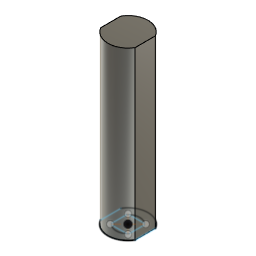
Joystick Extender (Autodesk Fusion 360 design; units mm, degrees)
Autodesk Fusion 360 part; units mm, degrees
sketch "Sketch1" plane through (0, 0, 0) normal (0, 0, 1) x (1, 0, 0)
  line L0 (1.3229, -1.5) -> (-1.3229, -1.5)
  line L1 (-1.5, -1.3229) -> (-1.5, 1.3229)
  line L2 (-1.3229, 1.5) -> (1.3229, 1.5)
  line L3 (1.5, 1.3229) -> (1.5, -1.3229)
  line L4 (1.5, -1.5) -> (-1.5, 1.5) construction
  line L5 (-1.5, -1.5) -> (1.5, 1.5) construction
  arc A0 (-1.5, -1.3229) -> (1.5, -1.3229) centre (0, 0) ccw
  arc A1 (1.5, 1.3229) -> (-1.5, 1.3229) centre (0, 0) ccw
  line L6 (-3, -1.8028) -> (-3, 1.8028)
  arc A2 (3, 1.8028) -> (-3, 1.8028) centre (0, 0) ccw
  line L7 (3, 1.8028) -> (3, -1.8028)
  arc A3 (-3, -1.8028) -> (3, -1.8028) centre (0, 0) ccw
  dimension "d1" = 4
  dimension "d2" = 3
  dimension "d3" = 3
  dimension "d4" = 1.5
  constraint coincident A0.centre A1.centre
  constraint horizontal L0
  constraint perpendicular L0 L1
  constraint parallel L0 L2
  constraint parallel L1 L3
  constraint coincident L4 A0.centre
  constraint coincident L5 A0.centre
  constraint coincident L2.start A0
  constraint coincident L0.end A0
  constraint coincident L3.start A0
  constraint coincident L2.end A0
  constraint coincident L0.start A0
  constraint concentric A0 A1
  measures "d1" diameter of A0
  measures "d2" distance of L4.end L5.end
  measures "d3" distance of L5.start L4.end
extrude "Extrude1" add sketch "Sketch1" along normal blind 30 contours L0 A0 | L0 L1 L2 L3 A0 A1 | L2 A1 | L6 A2 L7 A3 makes body 1
extrude "Extrude2" cut sketch "Sketch1" along normal blind 5 contours L0 A0 | L0 L1 L2 L3 A0 A1 | L2 A1 bodies 1
sketch "Sketch2" plane through (0, 0, 0) normal (0, 0, 1) x (1, 0, 0)
  line L0 (1.3601, -1.6) -> (-1.3601, -1.6)
  line L1 (-1.6, -1.3601) -> (-1.6, 1.3601)
  line L2 (-1.3601, 1.6) -> (1.3601, 1.6)
  line L3 (1.6, 1.3601) -> (1.6, -1.3601)
  line L4 (1.6, -1.6) -> (-1.6, 1.6) construction
  line L5 (-1.6, -1.6) -> (1.6, 1.6) construction
  arc A0 (-1.6, -1.3601) -> (1.6, -1.3601) centre (0, 0) ccw
  arc A1 (1.6, 1.3601) -> (-1.6, 1.3601) centre (0, 0) ccw
  line L6 (-3.1, -1.8303) -> (-3.1, 1.8303)
  arc A2 (3.1, 1.8303) -> (-3.1, 1.8303) centre (0, 0) ccw
  line L7 (3.1, 1.8303) -> (3.1, -1.8303)
  arc A3 (-3.1, -1.8303) -> (3.1, -1.8303) centre (0, 0) ccw
  dimension "d9" = 4.2
  dimension "d10" = 3.2
  dimension "d11" = 3.2
  dimension "d12" = 1.5
  constraint coincident A0.centre A1.centre
  constraint horizontal L0
  constraint perpendicular L0 L1
  constraint parallel L0 L2
  constraint parallel L1 L3
  constraint coincident L4 A0.centre
  constraint coincident L5 A0.centre
  constraint coincident L2.start A0
  constraint coincident L2.end A0
  constraint coincident L3.start A0
  constraint coincident L0.start A0
  constraint coincident L0.end A0
  constraint concentric A0 A1
  measures "d9" diameter of A0
  measures "d10" distance of L4.end L5.end
  measures "d11" distance of L5.start L4.end
extrude "Extrude3" add sketch "Sketch2" along normal blind 30 separate body contours L0 A0 | L0 L1 L2 L3 A0 A1 | L2 A1 | L6 A2 L7 A3 makes body 2
extrude "Extrude4" cut sketch "Sketch2" along normal blind 5 contours L0 A0 | L0 L1 L2 L3 A0 A1 | L2 A1 bodies 2
hidden bodies 1
